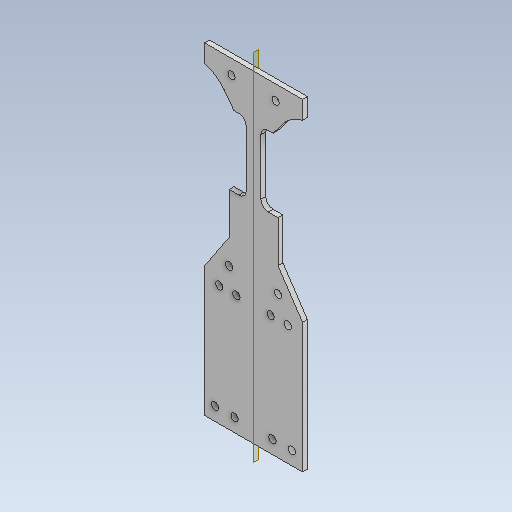
# Autodesk Inventor part: body_bone_5
Saved by Autodesk Inventor 2020 (Build 240168000, 168)
## iProperties
Created: 2019-05-16
Part Number: body_bone_5
Material: Generic
Document SubType Name: Modeling
Designer: psrob
Density: 1 g/cm^3
Appearance: Default
Author: psrob
Autodesk Inventor part; units mm, degrees
ref_plane "YZ Plane" through (0, 0, 0) normal (1, 0, 0) x (0, 1, 0)
ref_plane "XZ Plane" through (0, 0, 0) normal (0, 1, 0) x (-1, 0, 0)
ref_plane "XY Plane" through (0, 0, 0) normal (0, 0, 1) x (1, 0, 0)
sketch "Sketch1" plane through (0, 0, 0) normal (0, 0, 1) x (1, 0, 0)
  circle A0 centre (-14, 4) radius 1.5 projected
  circle A1 centre (-10, 13) radius 1.5 projected
  circle A2 centre (-7, 4) radius 1.5 projected
  line L0 (-20, 0) -> (-20, 8) projected
  line L1 (0, 0) -> (-20, 0) projected
  line L2 (0, 40) -> (0, 0) projected
  line L3 (-10, 40) -> (0, 40) projected
  line L4 (-10, 23) -> (-10, 40) projected
  line L5 (-10, 23) -> (-20, 8) projected
  circle A3 centre (14, 4) radius 1.5 projected
  circle A4 centre (10, 13) radius 1.5 projected
  circle A5 centre (7, 4) radius 1.5 projected
  line L6 (20, 0) -> (20, 8) projected
  line L7 (10, 23) -> (20, 8) projected
  line L8 (10, 23) -> (10, 40) projected
  line L9 (10, 40) -> (0, 40) projected
  line L10 (0, 40) -> (0, 0) projected
  line L11 (0, 0) -> (20, 0) projected
  arc A6 (-12.05, 74.2834) -> (-20, 79.501) centre (-23.25, 65.8834) ccw projected
  line L12 (-8.0217, 68.9123) -> (-12.05, 74.2834) projected
  line L13 (-10, 40) -> (-8.0217, 68.9123) projected
  line L14 (-10, 23) -> (-10, 40) projected
  line L15 (-20, 8) -> (-10, 23) projected
  line L16 (-20, -45) -> (-20, 8) projected
  line L17 (20, -45) -> (-20, -45) projected
  line L18 (20, 8) -> (20, -45) projected
  line L19 (10, 23) -> (20, 8) projected
  line L20 (10, 40) -> (10, 23) projected
  line L21 (8.0217, 68.9123) -> (10, 40) projected
  line L22 (12.05, 74.2834) -> (8.0217, 68.9123) projected
  arc A7 (20, 79.501) -> (12.05, 74.2834) centre (23.25, 65.8834) ccw projected
  line L23 (20, 86.8834) -> (20, 79.501) projected
  line L24 (-20, 86.8834) -> (20, 86.8834) projected
  line L25 (-20, 79.501) -> (-20, 86.8834) projected
  circle A8 centre (10, 13) radius 1.5 projected
  circle A9 centre (7, 4) radius 1.5 projected
  circle A10 centre (14, 4) radius 1.5 projected
  circle A11 centre (-14, 4) radius 1.5 projected
  circle A12 centre (-7, 4) radius 1.5 projected
  circle A13 centre (-10, 13) radius 1.5 projected
  circle A14 centre (9, 80.8834) radius 1.5 projected
  circle A15 centre (-9, 80.8834) radius 1.5 projected
  line L26 (3, 264.8834) -> (-3, 264.8834) projected
  line L27 (-3, 264.8834) -> (-3, -35.1166) projected
  line L28 (3, -35.1166) -> (-3, -35.1166) projected
  line L29 (3, 264.8834) -> (3, -35.1166) projected
  line L30 (8.0217, 68.9123) -> (-8.0217, 68.9123)
  line L31 (3, 40) -> (-3, 40)
  line L32 (-3, 40) -> (-3, 68.9123)
  line L33 (-3, 68.9123) -> (3, 68.9123)
  line L34 (3, 68.9123) -> (3, 40)
  circle A16 centre (-7.7386, -39.5) radius 1.5 projected
  circle A17 centre (-15.7386, -39.5) radius 1.5 projected
  circle A18 centre (7.7386, -39.5) radius 1.5 projected
  circle A19 centre (15.7386, -39.5) radius 1.5 projected
  point P0 (-3, 40)
  point P1 (3, 68.9123)
  constraints: 10 end point, 4 point on line, 2 horizontal, 2 parallel, 1 perpendicular
extrude "Extrusion1" add sketch "Sketch1" along normal blind 2 contours L0 L5 L4 L3 L27 L1 | L1 L27 L28 L29 L11 L18 L17 L16 | L27 L3 L2 L1 | L1 L11 L29 L28 L27 | L2 L9 L29 L11 | L27 L30 L29 L9 L3 | L29 L9 L8 L7 L6 L11 | L30 L12 A6 L25 L24 L27 | L27 L24 L29 L30 | L29 L24 L23 A7 L22 L30 | A16 | A17 | A18 | A19
fillet "Fillet1" radius 3 4 edges at (3, 40, 1) (-3, 40, 1) (-3, 68.9123, 1) (3, 68.9123, 1)
sketch "Sketch2" plane through (0, 0, 2) normal (0, 0, 1) x (1, 0, 0)
  circle A0 centre (-7.7386, -39.5) radius 1.5 projected
  circle A1 centre (-15.7386, -39.5) radius 1.5 projected
  point P0 (0, 0)
extrude "Extrusion2" cut sketch "Sketch2" against normal blind 10
ref_plane "Work Plane1" through (0, -45, 0) normal (-1, 0, 0) x (0, 0, 1)
mirror "Mirror1" about plane through (0, -45, 0) normal (-1, 0, 0) of "Extrusion2"
body "Solid1"
